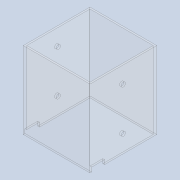
# Autodesk Inventor part: Part4_cover
Saved by Autodesk Inventor 2020 (Build 240168000, 168)
## iProperties
Created: 2019-05-16
Part Number: Part4_cover
Material: ABS Plastic
Document SubType Name: Modeling
Designer: kimhos
Density: 1.06 g/cm^3
Appearance: Clear - Light
Author: kimhos
Autodesk Inventor part; units mm, degrees
ref_plane "YZ Plane" through (0, 0, 0) normal (1, 0, 0) x (0, 1, 0)
ref_plane "XZ Plane" through (0, 0, 0) normal (0, 1, 0) x (-1, 0, 0)
ref_plane "XY Plane" through (0, 0, 0) normal (0, 0, 1) x (1, 0, 0)
sketch "Sketch1" plane through (0, 0, 0) normal (0, 1, 0) x (-1, 0, 0)
  line L0 (7.8, 0) -> (7.8, -7.8)
  line L1 (7.8, -7.8) -> (-7.8, -7.8)
  line L2 (-7.8, -7.8) -> (-7.8, 7.8)
  line L3 (-7.8, 7.8) -> (7.8, 7.8)
  line L4 (7.8, 7.8) -> (7.8, 0)
  line L5 (7.8, 7.8) -> (7, 7.8)
  line L6 (-7.8, 7.8) -> (-7.8, 7.4)
  line L7 (-7.8, -7.8) -> (-7.4, -7.8)
  line L8 (7.8, -7.8) -> (7.8, -7.4)
  line L9 (0, 0) -> (7.4, 0)
  line L10 (7.4, 0) -> (7.4, -7.4)
  line L11 (7.4, -7.4) -> (-7.4, -7.4)
  line L12 (-7.4, -7.4) -> (-7.4, 7.4)
  line L13 (-7.4, 7.4) -> (7.4, 7.4)
  line L14 (7.4, 7.4) -> (7.4, 0)
  line L15 (2.7947, -7.8) -> (2.7947, -7.4)
  dimension "d1" = 7.8
  dimension "d2" = 15.6
  dimension "d3" = 15.6
  dimension "d4" = 15.6
  dimension "d5" = 7.8
  dimension "d62" = 7.4
  dimension "d63" = 7.4
  dimension "d64" = 14.8
  dimension "d65" = 14.8
  dimension "d66" = 14.8
  dimension "d68" = 0.4
  constraints: 32 end point, 7 point on line, 6 perpendicular, 1 horizontal, 1 vertical
  measures "d1" distance of L0.start L0.end
  measures "d2" distance of L0.end L1.end
  measures "d3" distance of L1.end L2.end
  measures "d4" distance of L2.end L3.end
  measures "d5" distance of L3.end L0.start
  measures "d62" distance of L9.start L9.end
  measures "d63" distance of L9.end L10.end
  measures "d64" distance of L10.end L11.end
  measures "d65" distance of L11.end L12.end
  measures "d66" distance of L12.end L13.end
  measures "d68" distance of L15.start L15.end
extrude "Extrusion1" add sketch "Sketch1" along normal blind 18 contours L0 L1 L2 L3 L4 | L10 L11 L12 L13 L14
shell "Shell2" thickness 0.4 removed faces 2 at (2.6, 18, 0) at (2.6, 0, 0)
sketch "Sketch4" plane through (-7.8, 0, -7.8) normal (-1, 0, 0) x (0, 0, 1)
  line L0 (7.8, 0) -> (7.8, 4)
  circle A0 centre (7.8, 4) radius 0.5
  dimension "d17" = 4
  dimension "d18" = 1
  constraints: 2 end point, 1 centre point, 1 coincident, 1 vertical
  measures "d17" distance of L0.start L0.end
  measures "d18" diameter of A0
hole "Hole1" at (-7.8, 4, 0) direction (1, 0, 0) diameter 1 depth 20
sketch "Sketch8" plane through (7.8, 0, 7.8) normal (1, 0, 0) x (0, 0, -1)
  line L0 (15.2, 18) -> (0.4, 18) projected
  line L1 (7.8, 18) -> (7.8, 14)
  circle A0 centre (7.8, 14) radius 0.5
  point P0 (7.8, 0)
  dimension "d50" = 4
  dimension "d51" = 1
  constraints: 2 end point, 1 centre point, 1 coincident, 1 midpoint, 1 vertical
  measures "d50" distance of L1.start L1.end
  measures "d51" diameter of A0
hole "Hole4" at (7.8, 14, 0) direction (-1, 0, 0) diameter 1 depth 20
sketch "Sketch9" plane through (0, 0, 0) normal (0, -1, 0) x (1, 0, 0)
  line L0 (7.4, 7.4) -> (-7.4, 7.4) projected
  line L1 (-7.4, 7.4) -> (-7.4, 4.4)
  line L2 (-7.4, -7.4) -> (-7.4, 7.4) projected
  line L3 (-7.4, 4.4) -> (-7.8, 4.4)
  line L4 (-7.8, -7.8) -> (-7.8, 7.8) projected
  line L5 (-7.8, 4.4) -> (-7.8, 7.4)
  line L6 (-7.8, 7.4) -> (-7.4, 7.4)
  line L7 (7.4, 7.4) -> (7.4, 4.4)
  line L8 (7.4, 7.4) -> (7.4, -7.4) projected
  line L9 (7.4, 4.4) -> (7.8, 4.4)
  line L10 (7.8, 7.8) -> (7.8, -7.8) projected
  line L11 (7.8, 4.4) -> (7.8, 7.4)
  line L12 (7.8, 7.4) -> (7.4, 7.4)
  point P0 (0, 0)
  dimension "d69" = 3
  dimension "d70" = 3
  constraints: 16 end point, 6 point on line, 4 perpendicular
  measures "d69" distance of L0.end L1.end
  measures "d70" distance of L0.start L7.end
extrude "Extrusion2" cut sketch "Sketch9" against normal blind 1
body "Solid1"
